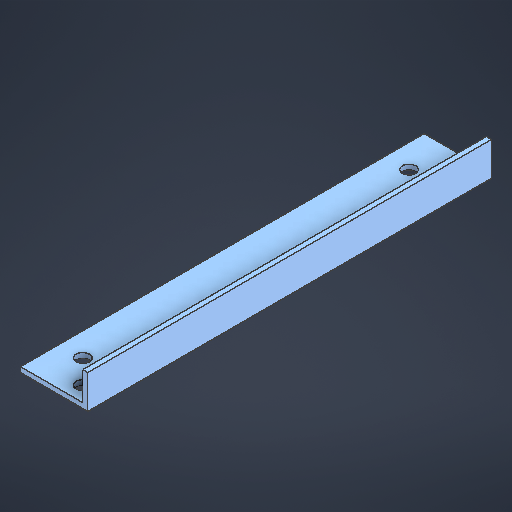
# Autodesk Inventor part: aluminium_profile_1
Saved by Autodesk Inventor 2026.1 (Build 301233000, 233)
## iProperties
Created: 2025-10-11
Part Number: aluminium_profile_1
Material: Generic
Document SubType Name: Modeling
Designer: emanuel
Density: 1 g/cm^3
Appearance: Default
Author: emanuel
Autodesk Inventor part; units mm, degrees
ref_plane "YZ Plane" through (0, 0, 0) normal (1, 0, 0) x (0, 1, 0)
ref_plane "XZ Plane" through (0, 0, 0) normal (0, 1, 0) x (-1, 0, 0)
ref_plane "XY Plane" through (0, 0, 0) normal (0, 0, 1) x (1, 0, 0)
sketch "Sketch1" plane through (0, 0, 0) normal (0, 1, 0) x (-1, 0, 0)
  line L0 (0, 0) -> (20, 0)
  line L1 (20, 0) -> (20, -120)
  line L2 (20, -120) -> (0, -120)
  line L3 (0, -120) -> (0, 0)
  dimension "d0" = 20
  dimension "d1" = 120
  constraints: 8 end point, 2 parallel, 1 horizontal, 1 perpendicular
  measures "d0" distance of L1.end L2.end
  measures "d1" distance of L0.end L1.end
extrude "Extrusion1" add sketch "Sketch1" along normal blind 1.5
sketch "Sketch2" plane through (0, 0, 0) normal (0, -1, 0) x (1, 0, 0)
  line L0 (0, 0) -> (-1.5, 0)
  line L1 (-1.5, 0) -> (-1.5, -120)
  line L2 (-1.5, -120) -> (0, -120)
  line L3 (0, -120) -> (0, 0)
  dimension "d4" = 1.5
  dimension "d5" = 120
  constraints: 8 end point, 2 parallel, 1 horizontal, 1 perpendicular
  measures "d4" distance of L2.end L1.end
  measures "d5" distance of L1.end L0.end
extrude "Extrusion2" add sketch "Sketch2" against normal blind 10
sketch "Sketch3" plane through (0, 1.5, 0) normal (0, 1, 0) x (1, 0, 0)
  line L0 (-20, 120) -> (-20, 0) projected
  line L1 (-20, 120) -> (-1.5, 120)
  line L2 (-1.5, 120) -> (-1.5, 101.5)
  line L3 (-1.5, 101.5) -> (-20, 101.5)
  line L4 (-20, 101.5) -> (-20, 120)
  line L5 (-20, 0) -> (-1.5, 0)
  line L6 (-1.5, 0) -> (-1.5, 18.5)
  line L7 (-1.5, 18.5) -> (-20, 18.5)
  line L8 (-20, 18.5) -> (-20, 0)
  line L9 (-20, 101.5) -> (-13, 101.5)
  line L10 (-13, 101.5) -> (-13, 108.5)
  line L11 (-13, 108.5) -> (-20, 108.5)
  line L12 (-20, 108.5) -> (-20, 101.5)
  line L13 (-20, 101.5) -> (-6, 101.5)
  line L14 (-6, 101.5) -> (-6, 115.5)
  line L15 (-6, 115.5) -> (-20, 115.5)
  line L16 (-20, 115.5) -> (-20, 101.5)
  circle A0 centre (-6, 115.5) radius 2
  circle A1 centre (-13, 108.5) radius 2
  line L17 (-20, 18.5) -> (-13, 18.5)
  line L18 (-13, 18.5) -> (-13, 11.5)
  line L19 (-13, 11.5) -> (-20, 11.5)
  line L20 (-20, 11.5) -> (-20, 18.5)
  line L21 (-20, 18.5) -> (-6, 18.5)
  line L22 (-6, 18.5) -> (-6, 4.5)
  line L23 (-6, 4.5) -> (-20, 4.5)
  line L24 (-20, 4.5) -> (-20, 18.5)
  circle A2 centre (-13, 11.5) radius 2
  circle A3 centre (-6, 4.5) radius 2
  point P0 (0, 0)
  dimension "d8" = 18.5
  dimension "d9" = 18.5
  dimension "d10" = 18.5
  dimension "d11" = 18.5
  dimension "d12" = 7
  dimension "d13" = 7
  dimension "d14" = 14
  dimension "d15" = 14
  dimension "d16" = 4
  dimension "d17" = 4
  dimension "d18" = 7
  dimension "d19" = 7
  dimension "d20" = 14
  dimension "d21" = 14
  dimension "d22" = 4
  dimension "d23" = 4
  constraints: 48 end point, 12 parallel, 6 horizontal, 6 perpendicular, 4 centre point, 4 coincident
  measures "d8" distance of L2.end L3.end
  measures "d9" distance of L1.end L2.end
  measures "d10" distance of L7.end L6.end
  measures "d11" distance of L6.end L5.end
  measures "d12" distance of L11.end L10.end
  measures "d13" distance of L10.end L9.end
  measures "d14" distance of L15.end L14.end
  measures "d15" distance of L14.end L13.end
  measures "d16" diameter of A0
  measures "d17" diameter of A1
  measures "d18" distance of L18.end L19.end
  measures "d19" distance of L17.end L18.end
  measures "d20" distance of L22.end L23.end
  measures "d21" distance of L21.end L22.end
  measures "d22" diameter of A2
  measures "d23" diameter of A3
extrude "Extrusion3" cut sketch "Sketch3" against normal blind 10 contours A0 L14 L15 | L15 L14 A0 | A1 L10 L11 | L11 L10 A1 | A2 L18 L19 | L19 L18 A2 | A3 L22 L23 | L23 L22 A3
body "Solid1"
